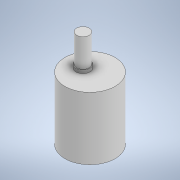
# Autodesk Inventor part: silnik
Saved by Autodesk Inventor 2022 (Build 260153000, 153)
## iProperties
Created: 2025-04-23
Part Number: silnik
Material: Ogólny
Document SubType Name: Modeling
Designer: Olga Kowalczyk IB 240875
Density: 1 g/cm^3
Appearance: Domyślna
Author: Olga Kowalczyk IB 240875
Autodesk Inventor part; units mm, degrees
ref_plane "YZ Plane" through (0, 0, 0) normal (1, 0, 0) x (0, 1, 0)
ref_plane "XZ Plane" through (0, 0, 0) normal (0, 1, 0) x (-1, 0, 0)
ref_plane "XY Plane" through (0, 0, 0) normal (0, 0, 1) x (1, 0, 0)
sketch "Szkic1" plane through (0, 0, 0) normal (0, 1, 0) x (-1, 0, 0)
  circle A0 centre (0, 0) radius 16
  circle A1 centre (4.5, 0) radius 4.5
  circle A2 centre (4.5, 0) radius 4
  dimension "d1" = 9
  dimension "d0" = 32
  dimension "d2" = 8
  constraints: 2 centre point, 2 coincident, 2 horizontal alignment, 2 other
  measures "d0" diameter of A0
  measures "d2" diameter of A2
extrude "Wyciągnięcie proste1" add sketch "Szkic1" along normal blind 40 contours A0
extrude "Wyciągnięcie proste2" add sketch "Szkic1" along normal blind 42 contours A1
extrude "Wyciągnięcie proste3" add sketch "Szkic1" along normal blind 60 contours A2
